Autodesk Fusion 360 part; units mm, degrees
note: some values were not read from the file. Set by a fixed rule: which sketch regions a step uses.
(part 20 of 59)
  spline S113 degree 5 poles (-3.9508, -16.2753) (-3.9508, -16.2754) (-3.9508, -16.2756) (-3.9509, -16.2759) (-3.9509, -16.2764) (-3.951, -16.2772) (-3.9511, -16.278) (-3.9512, -16.279) (-3.9514, -16.2801) (-3.9515, -16.2813) (-3.9517, -16.2826) (-3.9518, -16.284) (-3.952, -16.2855) (-3.9522, -16.2871) (-3.9523, -16.2889) (-3.9525, -16.2907) (-3.9527, -16.2926) (-3.9529, -16.2946) (-3.9531, -16.2968) (-3.9534, -16.299) (-3.9536, -16.3013) (-3.9538, -16.3037) (-3.954, -16.3063) (-3.9543, -16.3089) (-3.9545, -16.3116) (-3.9547, -16.3144) (-3.955, -16.3172) (-3.9552, -16.3202) (-3.9555, -16.3233) (-3.9557, -16.3264) (-3.9559, -16.3297) (-3.9562, -16.333) (-3.9564, -16.3364) (-3.9567, -16.3399) (-3.9569, -16.3435) (-3.9572, -16.3472) (-3.9574, -16.3509) (-3.9577, -16.3547) (-3.9579, -16.3586) (-3.9581, -16.3626) (-3.9584, -16.3667) (-3.9586, -16.3709) (-3.9588, -16.3751) (-3.959, -16.3794) (-3.9593, -16.3838) (-3.9595, -16.3882) (-3.9597, -16.3928) (-3.9599, -16.3974) (-3.9601, -16.4021) (-3.9603, -16.4068) (-3.9605, -16.4117) (-3.9607, -16.4166) (-3.9609, -16.4215) (-3.961, -16.4266) (-3.9612, -16.4317) (-3.9614, -16.4369) (-3.9615, -16.4422) (-3.9617, -16.4475) (-3.9618, -16.4529) (-3.962, -16.4584) (-3.9621, -16.4639) (-3.9622, -16.4695) (-3.9623, -16.4752) (-3.9624, -16.4809) (-3.9625, -16.4867) (-3.9626, -16.4926) (-3.9627, -16.4985) (-3.9627, -16.5045) (-3.9628, -16.5106) (-3.9629, -16.5167) (-3.9629, -16.5229) (-3.9629, -16.5291) (-3.9629, -16.5355) (-3.963, -16.5418) (-3.963, -16.5483) (-3.9629, -16.5548) (-3.9629, -16.5613) (-3.9629, -16.568) (-3.9628, -16.5746) (-3.9628, -16.5814) (-3.9627, -16.5882) (-3.9626, -16.595) (-3.9626, -16.6019) (-3.9625, -16.6089) (-3.9623, -16.6159) (-3.9622, -16.623) (-3.9621, -16.6302) (-3.9619, -16.6374) (-3.9618, -16.6446) (-3.9616, -16.6519) (-3.9614, -16.6593) (-3.9612, -16.6667) (-3.961, -16.6742) (-3.9607, -16.6817) (-3.9605, -16.6893) (-3.9603, -16.697) (-3.96, -16.7047) (-3.9597, -16.7124) (-3.9594, -16.7202) (-3.9591, -16.7281) (-3.9588, -16.736) (-3.9584, -16.7439) (-3.9581, -16.7519) (-3.9577, -16.76) (-3.9573, -16.7681) (-3.9569, -16.7763) (-3.9565, -16.7845) (-3.9561, -16.7927) (-3.9556, -16.801) (-3.9552, -16.8094) (-3.9547, -16.8178) (-3.9542, -16.8263) (-3.9537, -16.8348) (-3.9532, -16.8433) (-3.9526, -16.8519) (-3.9521, -16.8606) (-3.9515, -16.8693) (-3.9509, -16.878) (-3.9503, -16.8868) (-3.9497, -16.8957) (-3.9491, -16.9045) (-3.9484, -16.9135) (-3.9478, -16.9225) (-3.9471, -16.9315) (-3.9464, -16.9406) (-3.9457, -16.9497) (-3.9449, -16.9588) (-3.9442, -16.968) (-3.9434, -16.9773) (-3.9426, -16.9866) (-3.9418, -16.9959) (-3.941, -17.0053) (-3.9402, -17.0147) (-3.9393, -17.0242) (-3.9384, -17.0337) (-3.9375, -17.0433) (-3.9366, -17.0529) (-3.9357, -17.0625) (-3.9348, -17.0722) (-3.9338, -17.0819) (-3.9328, -17.0917) (-3.9318, -17.1015) (-3.9308, -17.1113) (-3.9297, -17.1212) (-3.9287, -17.1312) (-3.9276, -17.1411) (-3.9265, -17.1512) (-3.9254, -17.1612) (-3.9243, -17.1713) (-3.9231, -17.1814) (-3.922, -17.1916) (-3.9208, -17.2018) (-3.9196, -17.2121) (-3.9183, -17.2224) (-3.9171, -17.2327) (-3.9158, -17.2431) (-3.9145, -17.2535) (-3.9132, -17.264) (-3.9119, -17.2744) (-3.9106, -17.285) (-3.9092, -17.2955) (-3.9078, -17.3061) (-3.9064, -17.3168) (-3.905, -17.3274) (-3.9035, -17.3382) (-3.9021, -17.3489) (-3.9006, -17.3597) (-3.8991, -17.3705) (-3.8976, -17.3814) (-3.896, -17.3923) (-3.8945, -17.4032) (-3.8929, -17.4142) (-3.8913, -17.4252) (-3.8896, -17.4362) (-3.888, -17.4473) (-3.8863, -17.4584) (-3.8846, -17.4696) (-3.8829, -17.4807) (-3.8812, -17.492) (-3.8795, -17.5032) (-3.8777, -17.5145) (-3.8759, -17.5258) (-3.8741, -17.5372) (-3.8722, -17.5486) (-3.8704, -17.56) (-3.8685, -17.5714) (-3.8666, -17.5829) (-3.8647, -17.5944) (-3.8628, -17.606) (-3.8608, -17.6176) (-3.8588, -17.6292) (-3.8568, -17.6409) (-3.8548, -17.6525) (-3.8527, -17.6643) (-3.8507, -17.676) (-3.8486, -17.6878) (-3.8464, -17.6996) (-3.8443, -17.7115) (-3.8422, -17.7233) (-3.84, -17.7353) (-3.8378, -17.7472) (-3.8356, -17.7592) (-3.8333, -17.7712) (-3.831, -17.7832) (-3.8288, -17.7953) (-3.8264, -17.8074) (-3.8241, -17.8195) (-3.8217, -17.8317) (-3.8194, -17.8439) (-3.817, -17.8561) (-3.8145, -17.8683) (-3.8121, -17.8806) (-3.8096, -17.8929) (-3.8071, -17.9053) (-3.8046, -17.9176) (-3.8021, -17.93) (-3.7995, -17.9424) (-3.797, -17.9549) (-3.7943, -17.9674) (-3.7917, -17.9799) (-3.7891, -17.9924) (-3.7864, -18.005) (-3.7837, -18.0176) (-3.781, -18.0302) (-3.7782, -18.0429) (-3.7755, -18.0556) (-3.7727, -18.0683) (-3.7699, -18.081) (-3.767, -18.0938) (-3.7642, -18.1066) (-3.7613, -18.1194) (-3.7584, -18.1323) (-3.7555, -18.1451) (-3.7525, -18.158) (-3.7496, -18.171) (-3.7466, -18.1839) (-3.7435, -18.1969) (-3.7405, -18.2099) (-3.7374, -18.223) (-3.7343, -18.236) (-3.7312, -18.2491) (-3.7287, -18.2596) (-3.7268, -18.2675) (-3.7256, -18.2728) (-3.7249, -18.2754) knots 0 0 0 0 0 0 0.00416667 0.00833333 0.0125 0.01666667 0.02083333 0.025 0.02916667 0.03333333 0.0375 0.04166667 0.04583333 0.05 0.05416667 0.05833333 0.0625 0.06666667 0.07083333 0.075 0.07916667 0.08333333 0.0875 0.09166667 0.09583333 0.1 0.10416667 0.10833333 0.1125 0.11666667 0.12083333 0.125 0.12916667 0.13333333 0.1375 0.14166667 0.14583333 0.15 0.15416667 0.15833333 0.1625 0.16666667 0.17083333 0.175 0.17916667 0.18333333 0.1875 0.19166667 0.19583333 0.2 0.20416667 0.20833333 0.2125 0.21666667 0.22083333 0.225 0.22916667 0.23333333 0.2375 0.24166667 0.24583333 0.25 0.25416667 0.25833333 0.2625 0.26666667 0.27083333 0.275 0.27916667 0.28333333 0.2875 0.29166667 0.29583333 0.3 0.30416667 0.30833333 0.3125 0.31666667 0.32083333 0.325 0.32916667 0.33333333 0.3375 0.34166667 0.34583333 0.35 0.35416667 0.35833333 0.3625 0.36666667 0.37083333 0.375 0.37916667 0.38333333 0.3875 0.39166667 0.39583333 0.4 0.40416667 0.40833333 0.4125 0.41666667 0.42083333 0.425 0.42916667 0.43333333 0.4375 0.44166667 0.44583333 0.45 0.45416667 0.45833333 0.4625 0.46666667 0.47083333 0.475 0.47916667 0.48333333 0.4875 0.49166667 0.49583333 0.5 0.50416667 0.50833333 0.5125 0.51666667 0.52083333 0.525 0.52916667 0.53333333 0.5375 0.54166667 0.54583333 0.55 0.55416667 0.55833333 0.5625 0.56666667 0.57083333 0.575 0.57916667 0.58333333 0.5875 0.59166667 0.59583333 0.6 0.60416667 0.60833333 0.6125 0.61666667 0.62083333 0.625 0.62916667 0.63333333 0.6375 0.64166667 0.64583333 0.65 0.65416667 0.65833333 0.6625 0.66666667 0.67083333 0.675 0.67916667 0.68333333 0.6875 0.69166667 0.69583333 0.7 0.70416667 0.70833333 0.7125 0.71666667 0.72083333 0.725 0.72916667 0.73333333 0.7375 0.74166667 0.74583333 0.75 0.75416667 0.75833333 0.7625 0.76666667 0.77083333 0.775 0.77916667 0.78333333 0.7875 0.79166667 0.79583333 0.8 0.80416667 0.80833333 0.8125 0.81666667 0.82083333 0.825 0.82916667 0.83333333 0.8375 0.84166667 0.84583333 0.85 0.85416667 0.85833333 0.8625 0.86666667 0.87083333 0.875 0.87916667 0.88333333 0.8875 0.89166667 0.89583333 0.9 0.90416667 0.90833333 0.9125 0.91666667 0.92083333 0.925 0.92916667 0.93333333 0.9375 0.94166667 0.94583333 0.95 0.95416667 0.95833333 0.9625 0.96666667 0.97083333 0.975 0.97916667 0.98333333 0.9875 0.99166667 0.99583333 1 1 1 1 1 1
  line L242 (18.7406, 34.6904) -> (18.7401, 34.6898)
  line L243 (3.9507, 41.2745) -> (3.9508, 41.2753)
  spline S114 degree 5 poles (8.0948, -15.3945) (8.0948, -15.3946) (8.0948, -15.3948) (8.0949, -15.3951) (8.0951, -15.3956) (8.0953, -15.3963) (8.0956, -15.3971) (8.0958, -15.398) (8.0962, -15.3991) (8.0965, -15.4002) (8.0969, -15.4015) (8.0973, -15.4028) (8.0978, -15.4043) (8.0983, -15.4058) (8.0988, -15.4075) (8.0994, -15.4092) (8.1, -15.4111) (8.1007, -15.413) (8.1013, -15.415) (8.102, -15.4172) (8.1028, -15.4194) (8.1036, -15.4217) (8.1044, -15.4241) (8.1052, -15.4265) (8.1061, -15.4291) (8.107, -15.4318) (8.108, -15.4345) (8.109, -15.4373) (8.11, -15.4402) (8.1111, -15.4432) (8.1121, -15.4462) (8.1133, -15.4494) (8.1144, -15.4526) (8.1156, -15.4559) (8.1169, -15.4593) (8.1181, -15.4627) (8.1194, -15.4662) (8.1208, -15.4698) (8.1222, -15.4735) (8.1236, -15.4772) (8.125, -15.4811) (8.1265, -15.4849) (8.128, -15.4889) (8.1295, -15.4929) (8.1311, -15.497) (8.1327, -15.5012) (8.1344, -15.5054) (8.1361, -15.5097) (8.1378, -15.5141) (8.1395, -15.5185) (8.1413, -15.523) (8.1432, -15.5276) (8.145, -15.5322) (8.1469, -15.5369) (8.1488, -15.5416) (8.1508, -15.5464) (8.1528, -15.5513) (8.1548, -15.5562) (8.1569, -15.5612) (8.159, -15.5663) (8.1611, -15.5714) (8.1633, -15.5765) (8.1655, -15.5818) (8.1677, -15.587) (8.17, -15.5924) (8.1723, -15.5978) (8.1747, -15.6032) (8.177, -15.6087) (8.1795, -15.6143) (8.1819, -15.6199) (8.1844, -15.6256) (8.1869, -15.6313) (8.1895, -15.6371) (8.192, -15.6429) (8.1947, -15.6488) (8.1973, -15.6547) (8.2, -15.6607) (8.2027, -15.6667) (8.2055, -15.6728) (8.2083, -15.679) (8.2111, -15.6851) (8.214, -15.6914) (8.2169, -15.6977) (8.2198, -15.704) (8.2227, -15.7104) (8.2257, -15.7168) (8.2288, -15.7233) (8.2318, -15.7298) (8.2349, -15.7363) (8.2381, -15.7429) (8.2412, -15.7496) (8.2445, -15.7563) (8.2477, -15.763) (8.251, -15.7698) (8.2543, -15.7767) (8.2576, -15.7835) (8.261, -15.7905) (8.2644, -15.7974) (8.2678, -15.8044) (8.2713, -15.8115) (8.2748, -15.8186) (8.2784, -15.8257) (8.282, -15.8329) (8.2856, -15.8401) (8.2892, -15.8473) (8.2929, -15.8546) (8.2966, -15.8619) (8.3004, -15.8693) (8.3042, -15.8767) (8.308, -15.8842) (8.3118, -15.8917) (8.3157, -15.8992) (8.3196, -15.9068) (8.3236, -15.9144) (8.3276, -15.922) (8.3316, -15.9297) (8.3357, -15.9374) (8.3398, -15.9452) (8.3439, -15.9529) (8.348, -15.9608) (8.3522, -15.9686) (8.3565, -15.9765) (8.3607, -15.9845) (8.365, -15.9924) (8.3693, -16.0004) (8.3737, -16.0085) (8.3781, -16.0165) (8.3825, -16.0246) (8.387, -16.0328) (8.3915, -16.0409) (8.396, -16.0491) (8.4006, -16.0574) (8.4052, -16.0657) (8.4098, -16.074) (8.4145, -16.0823) (8.4192, -16.0907) (8.4239, -16.0991) (8.4287, -16.1075) (8.4335, -16.116) (8.4384, -16.1244) (8.4432, -16.133) (8.4481, -16.1415) (8.4531, -16.1501) (8.458, -16.1587) (8.463, -16.1674) (8.4681, -16.176) (8.4732, -16.1847) (8.4783, -16.1935) (8.4834, -16.2022) (8.4886, -16.211) (8.4938, -16.2199) (8.499, -16.2287) (8.5043, -16.2376) (8.5096, -16.2465) (8.515, -16.2554) (8.5203, -16.2644) (8.5257, -16.2734) (8.5312, -16.2824) (8.5367, -16.2914) (8.5422, -16.3005) (8.5477, -16.3096) (8.5533, -16.3187) (8.5589, -16.3279) (8.5645, -16.337) (8.5702, -16.3462) (8.5759, -16.3555) (8.5817, -16.3647) (8.5874, -16.374) (8.5932, -16.3833) (8.5991, -16.3926) (8.605, -16.402) (8.6109, -16.4113) (8.6168, -16.4207) (8.6228, -16.4302) (8.6288, -16.4396) (8.6348, -16.4491) (8.6409, -16.4586) (8.647, -16.4681) (8.6532, -16.4776) (8.6593, -16.4872) (8.6656, -16.4968) (8.6718, -16.5064) (8.6781, -16.516) (8.6844, -16.5257) (8.6907, -16.5354) (8.6971, -16.5451) (8.7035, -16.5548) (8.7099, -16.5646) (8.7164, -16.5743) (8.7229, -16.5841) (8.7295, -16.5939) (8.736, -16.6037) (8.7426, -16.6136) (8.7493, -16.6235) (8.7559, -16.6334) (8.7626, -16.6433) (8.7694, -16.6532) (8.7762, -16.6632) (8.783, -16.6731) (8.7898, -16.6831) (8.7967, -16.6932) (8.8036, -16.7032) (8.8105, -16.7132) (8.8175, -16.7233) (8.8245, -16.7334) (8.8315, -16.7435) (8.8386, -16.7537) (8.8457, -16.7638) (8.8528, -16.774) (8.86, -16.7842) (8.8671, -16.7944) (8.8744, -16.8046) (8.8816, -16.8148) (8.8889, -16.8251) (8.8963, -16.8354) (8.9036, -16.8457) (8.911, -16.856) (8.9184, -16.8663) (8.9259, -16.8766) (8.9334, -16.887) (8.9409, -16.8974) (8.9485, -16.9078) (8.956, -16.9182) (8.9637, -16.9286) (8.9713, -16.9391) (8.979, -16.9495) (8.9867, -16.96) (8.9945, -16.9705) (9.0022, -16.981) (9.0101, -16.9915) (9.0179, -17.0021) (9.0258, -17.0127) (9.0337, -17.0232) (9.0416, -17.0338) (9.0496, -17.0444) (9.0576, -17.055) (9.0657, -17.0657) (9.0737, -17.0763) (9.0818, -17.087) (9.09, -17.0977) (9.0981, -17.1084) (9.1047, -17.1169) (9.1096, -17.1234) (9.1129, -17.1276) (9.1146, -17.1298) knots 0 0 0 0 0 0 0.00416667 0.00833333 0.0125 0.01666667 0.02083333 0.025 0.02916667 0.03333333 0.0375 0.04166667 0.04583333 0.05 0.05416667 0.05833333 0.0625 0.06666667 0.07083333 0.075 0.07916667 0.08333333 0.0875 0.09166667 0.09583333 0.1 0.10416667 0.10833333 0.1125 0.11666667 0.12083333 0.125 0.12916667 0.13333333 0.1375 0.14166667 0.14583333 0.15 0.15416667 0.15833333 0.1625 0.16666667 0.17083333 0.175 0.17916667 0.18333333 0.1875 0.19166667 0.19583333 0.2 0.20416667 0.20833333 0.2125 0.21666667 0.22083333 0.225 0.22916667 0.23333333 0.2375 0.24166667 0.24583333 0.25 0.25416667 0.25833333 0.2625 0.26666667 0.27083333 0.275 0.27916667 0.28333333 0.2875 0.29166667 0.29583333 0.3 0.30416667 0.30833333 0.3125 0.31666667 0.32083333 0.325 0.32916667 0.33333333 0.3375 0.34166667 0.34583333 0.35 0.35416667 0.35833333 0.3625 0.36666667 0.37083333 0.375 0.37916667 0.38333333 0.3875 0.39166667 0.39583333 0.4 0.40416667 0.40833333 0.4125 0.41666667 0.42083333 0.425 0.42916667 0.43333333 0.4375 0.44166667 0.44583333 0.45 0.45416667 0.45833333 0.4625 0.46666667 0.47083333 0.475 0.47916667 0.48333333 0.4875 0.49166667 0.49583333 0.5 0.50416667 0.50833333 0.5125 0.51666667 0.52083333 0.525 0.52916667 0.53333333 0.5375 0.54166667 0.54583333 0.55 0.55416667 0.55833333 0.5625 0.56666667 0.57083333 0.575 0.57916667 0.58333333 0.5875 0.59166667 0.59583333 0.6 0.60416667 0.60833333 0.6125 0.61666667 0.62083333 0.625 0.62916667 0.63333333 0.6375 0.64166667 0.64583333 0.65 0.65416667 0.65833333 0.6625 0.66666667 0.67083333 0.675 0.67916667 0.68333333 0.6875 0.69166667 0.69583333 0.7 0.70416667 0.70833333 0.7125 0.71666667 0.72083333 0.725 0.72916667 0.73333333 0.7375 0.74166667 0.74583333 0.75 0.75416667 0.75833333 0.7625 0.76666667 0.77083333 0.775 0.77916667 0.78333333 0.7875 0.79166667 0.79583333 0.8 0.80416667 0.80833333 0.8125 0.81666667 0.82083333 0.825 0.82916667 0.83333333 0.8375 0.84166667 0.84583333 0.85 0.85416667 0.85833333 0.8625 0.86666667 0.87083333 0.875 0.87916667 0.88333333 0.8875 0.89166667 0.89583333 0.9 0.90416667 0.90833333 0.9125 0.91666667 0.92083333 0.925 0.92916667 0.93333333 0.9375 0.94166667 0.94583333 0.95 0.95416667 0.95833333 0.9625 0.96666667 0.97083333 0.975 0.97916667 0.98333333 0.9875 0.99166667 0.99583333 1 1 1 1 1 1
  arc A121 (-5.0824, -15.7972) -> (-3.9106, -15.9828) centre (0, 12.5) ccw
  line L244 (28.587, 17.6345) -> (28.5878, 17.6346)
  spline S115 degree 5 poles (6.937, 40.7047) (6.937, 40.7048) (6.937, 40.705) (6.9371, 40.7053) (6.9372, 40.7058) (6.9374, 40.7065) (6.9376, 40.7074) (6.9378, 40.7083) (6.9381, 40.7094) (6.9383, 40.7106) (6.9386, 40.7118) (6.9389, 40.7132) (6.9392, 40.7147) (6.9396, 40.7163) (6.9399, 40.718) (6.9403, 40.7198) (6.9407, 40.7217) (6.9411, 40.7237) (6.9416, 40.7258) (6.942, 40.728) (6.9425, 40.7303) (6.9429, 40.7327) (6.9434, 40.7351) (6.9439, 40.7377) (6.9445, 40.7404) (6.945, 40.7431) (6.9455, 40.746) (6.9461, 40.7489) (6.9466, 40.7519) (6.9472, 40.755) (6.9478, 40.7582) (6.9484, 40.7615) (6.949, 40.7649) (6.9496, 40.7683) (6.9502, 40.7719) (6.9508, 40.7755) (6.9515, 40.7792) (6.9521, 40.783) (6.9528, 40.7868) (6.9534, 40.7908) (6.9541, 40.7948) (6.9547, 40.7989) (6.9554, 40.8031) (6.9561, 40.8074) (6.9568, 40.8117) (6.9574, 40.8161) (6.9581, 40.8206) (6.9588, 40.8252) (6.9595, 40.8298) (6.9602, 40.8345) (6.9609, 40.8393) (6.9616, 40.8442) (6.9623, 40.8491) (6.963, 40.8541) (6.9637, 40.8592) (6.9644, 40.8643) (6.9651, 40.8695) (6.9658, 40.8748) (6.9665, 40.8802) (6.9672, 40.8856) (6.9679, 40.8911) (6.9686, 40.8966) (6.9693, 40.9023) (6.97, 40.908) (6.9707, 40.9137) (6.9714, 40.9196) (6.9721, 40.9255) (6.9728, 40.9314) (6.9735, 40.9374) (6.9742, 40.9435) (6.9749, 40.9497) (6.9756, 40.9559) (6.9763, 40.9622) (6.9769, 40.9685) (6.9776, 40.9749) (6.9783, 40.9814) (6.9789, 40.9879) (6.9796, 40.9945) (6.9803, 41.0011) (6.9809, 41.0078) (6.9816, 41.0146) (6.9822, 41.0214) (6.9828, 41.0283) (6.9835, 41.0353) (6.9841, 41.0423) (6.9847, 41.0493) (6.9853, 41.0564) (6.9859, 41.0636) (6.9865, 41.0709) (6.9871, 41.0781) (6.9877, 41.0855) (6.9882, 41.0929) (6.9888, 41.1004) (6.9894, 41.1079) (6.9899, 41.1154) (6.9905, 41.1231) (6.991, 41.1307) (6.9915, 41.1385) (6.9921, 41.1463) (6.9926, 41.1541) (6.9931, 41.162) (6.9936, 41.17) (6.994, 41.178) (6.9945, 41.186) (6.995, 41.1941) (6.9954, 41.2023) (6.9959, 41.2105) (6.9963, 41.2187) (6.9968, 41.227) (6.9972, 41.2354) (6.9976, 41.2438) (6.998, 41.2523) (6.9984, 41.2608) (6.9987, 41.2694) (6.9991, 41.278) (6.9995, 41.2866) (6.9998, 41.2953) (7.0001, 41.3041) (7.0005, 41.3129) (7.0008, 41.3218) (7.0011, 41.3307) (7.0014, 41.3396) (7.0016, 41.3486) (7.0019, 41.3577) (7.0021, 41.3668) (7.0024, 41.3759) (7.0026, 41.3851) (7.0028, 41.3943) (7.003, 41.4036) (7.0032, 41.4129) (7.0034, 41.4223) (7.0036, 41.4317) (7.0037, 41.4412) (7.0038, 41.4507) (7.004, 41.4602) (7.0041, 41.4698) (7.0042, 41.4795) (7.0043, 41.4892) (7.0043, 41.4989) (7.0044, 41.5087) (7.0044, 41.5185) (7.0045, 41.5284) (7.0045, 41.5383) (7.0045, 41.5482) (7.0045, 41.5582) (7.0044, 41.5682) (7.0044, 41.5783) (7.0043, 41.5884) (7.0043, 41.5986) (7.0042, 41.6088) (7.0041, 41.619) (7.004, 41.6293) (7.0038, 41.6396) (7.0037, 41.65) (7.0035, 41.6604) (7.0034, 41.6708) (7.0032, 41.6813) (7.003, 41.6919) (7.0028, 41.7024) (7.0025, 41.713) (7.0023, 41.7237) (7.002, 41.7344) (7.0017, 41.7451) (7.0014, 41.7559) (7.0011, 41.7667) (7.0008, 41.7775) (7.0004, 41.7884) (7.0001, 41.7993) (6.9997, 41.8103) (6.9993, 41.8213) (6.9989, 41.8323) (6.9984, 41.8434) (6.998, 41.8545) (6.9975, 41.8657) (6.997, 41.8768) (6.9965, 41.8881) (6.996, 41.8993) (6.9955, 41.9106) (6.995, 41.922) (6.9944, 41.9333) (6.9938, 41.9447) (6.9932, 41.9562) (6.9926, 41.9677) (6.992, 41.9792) (6.9913, 41.9907) (6.9906, 42.0023) (6.99, 42.014) (6.9892, 42.0256) (6.9885, 42.0373) (6.9878, 42.049) (6.987, 42.0608) (6.9863, 42.0726) (6.9855, 42.0844) (6.9846, 42.0963) (6.9838, 42.1082) (6.983, 42.1201) (6.9821, 42.1321) (6.9812, 42.1441) (6.9803, 42.1562) (6.9794, 42.1682) (6.9784, 42.1803) (6.9775, 42.1925) (6.9765, 42.2047) (6.9755, 42.2169) (6.9745, 42.2291) (6.9735, 42.2414) (6.9724, 42.2537) (6.9713, 42.266) (6.9702, 42.2784) (6.9691, 42.2908) (6.968, 42.3032) (6.9669, 42.3157) (6.9657, 42.3282) (6.9645, 42.3407) (6.9633, 42.3533) (6.9621, 42.3659) (6.9608, 42.3785) (6.9596, 42.3912) (6.9583, 42.4039) (6.957, 42.4166) (6.9556, 42.4293) (6.9543, 42.4421) (6.9529, 42.4549) (6.9516, 42.4678) (6.9501, 42.4806) (6.9487, 42.4935) (6.9473, 42.5065) (6.9458, 42.5194) (6.9443, 42.5324) (6.9428, 42.5455) (6.9413, 42.5585) (6.9398, 42.5716) (6.9382, 42.5847) (6.9366, 42.5979) (6.935, 42.611) (6.9334, 42.6242) (6.9317, 42.6375) (6.9301, 42.6507) (6.9284, 42.664) (6.9267, 42.6773) (6.925, 42.6907) (6.9236, 42.7014) (6.9225, 42.7094) (6.9218, 42.7148) (6.9214, 42.7174) knots 0 0 0 0 0 0 0.00416667 0.00833333 0.0125 0.01666667 0.02083333 0.025 0.02916667 0.03333333 0.0375 0.04166667 0.04583333 0.05 0.05416667 0.05833333 0.0625 0.06666667 0.07083333 0.075 0.07916667 0.08333333 0.0875 0.09166667 0.09583333 0.1 0.10416667 0.10833333 0.1125 0.11666667 0.12083333 0.125 0.12916667 0.13333333 0.1375 0.14166667 0.14583333 0.15 0.15416667 0.15833333 0.1625 0.16666667 0.17083333 0.175 0.17916667 0.18333333 0.1875 0.19166667 0.19583333 0.2 0.20416667 0.20833333 0.2125 0.21666667 0.22083333 0.225 0.22916667 0.23333333 0.2375 0.24166667 0.24583333 0.25 0.25416667 0.25833333 0.2625 0.26666667 0.27083333 0.275 0.27916667 0.28333333 0.2875 0.29166667 0.29583333 0.3 0.30416667 0.30833333 0.3125 0.31666667 0.32083333 0.325 0.32916667 0.33333333 0.3375 0.34166667 0.34583333 0.35 0.35416667 0.35833333 0.3625 0.36666667 0.37083333 0.375 0.37916667 0.38333333 0.3875 0.39166667 0.39583333 0.4 0.40416667 0.40833333 0.4125 0.41666667 0.42083333 0.425 0.42916667 0.43333333 0.4375 0.44166667 0.44583333 0.45 0.45416667 0.45833333 0.4625 0.46666667 0.47083333 0.475 0.47916667 0.48333333 0.4875 0.49166667 0.49583333 0.5 0.50416667 0.50833333 0.5125 0.51666667 0.52083333 0.525 0.52916667 0.53333333 0.5375 0.54166667 0.54583333 0.55 0.55416667 0.55833333 0.5625 0.56666667 0.57083333 0.575 0.57916667 0.58333333 0.5875 0.59166667 0.59583333 0.6 0.60416667 0.60833333 0.6125 0.61666667 0.62083333 0.625 0.62916667 0.63333333 0.6375 0.64166667 0.64583333 0.65 0.65416667 0.65833333 0.6625 0.66666667 0.67083333 0.675 0.67916667 0.68333333 0.6875 0.69166667 0.69583333 0.7 0.70416667 0.70833333 0.7125 0.71666667 0.72083333 0.725 0.72916667 0.73333333 0.7375 0.74166667 0.74583333 0.75 0.75416667 0.75833333 0.7625 0.76666667 0.77083333 0.775 0.77916667 0.78333333 0.7875 0.79166667 0.79583333 0.8 0.80416667 0.80833333 0.8125 0.81666667 0.82083333 0.825 0.82916667 0.83333333 0.8375 0.84166667 0.84583333 0.85 0.85416667 0.85833333 0.8625 0.86666667 0.87083333 0.875 0.87916667 0.88333333 0.8875 0.89166667 0.89583333 0.9 0.90416667 0.90833333 0.9125 0.91666667 0.92083333 0.925 0.92916667 0.93333333 0.9375 0.94166667 0.94583333 0.95 0.95416667 0.95833333 0.9625 0.96666667 0.97083333 0.975 0.97916667 0.98333333 0.9875 0.99166667 0.99583333 1 1 1 1 1 1
  spline S116 degree 5 poles (29.0307, 11.5787) (29.0307, 11.5787) (29.0309, 11.5787) (29.0313, 11.5787) (29.0318, 11.5787) (29.0325, 11.5787) (29.0334, 11.5787) (29.0344, 11.5786) (29.0355, 11.5786) (29.0367, 11.5786) (29.038, 11.5786) (29.0394, 11.5786) (29.0409, 11.5786) (29.0425, 11.5786) (29.0443, 11.5786) (29.0461, 11.5786) (29.0481, 11.5786) (29.0501, 11.5786) (29.0522, 11.5786) (29.0545, 11.5786) (29.0568, 11.5786) (29.0592, 11.5787) (29.0618, 11.5787) (29.0644, 11.5788) (29.0671, 11.5788) (29.0699, 11.5789) (29.0728, 11.5789) (29.0758, 11.579) (29.0788, 11.5791) (29.082, 11.5792) (29.0852, 11.5792) (29.0886, 11.5794) (29.092, 11.5795) (29.0955, 11.5796) (29.0991, 11.5797) (29.1028, 11.5799) (29.1065, 11.58) (29.1103, 11.5802) (29.1143, 11.5803) (29.1183, 11.5805) (29.1223, 11.5807) (29.1265, 11.5809) (29.1307, 11.5811) (29.135, 11.5814) (29.1394, 11.5816) (29.1439, 11.5818) (29.1484, 11.5821) (29.153, 11.5824) (29.1577, 11.5827) (29.1624, 11.583) (29.1673, 11.5833) (29.1722, 11.5836) (29.1771, 11.5839) (29.1822, 11.5843) (29.1873, 11.5847) (29.1925, 11.585) (29.1977, 11.5854) (29.203, 11.5859) (29.2084, 11.5863) (29.2139, 11.5867) (29.2194, 11.5872) (29.225, 11.5876) (29.2306, 11.5881) (29.2363, 11.5886) (29.2421, 11.5891) (29.248, 11.5897) (29.2539, 11.5902) (29.2599, 11.5908) (29.2659, 11.5913) (29.272, 11.5919) (29.2781, 11.5925) (29.2844, 11.5932) (29.2906, 11.5938) (29.297, 11.5945) (29.3034, 11.5951) (29.3099, 11.5958) (29.3164, 11.5965) (29.323, 11.5973) (29.3296, 11.598) (29.3363, 11.5988) (29.343, 11.5995) (29.3498, 11.6003) (29.3567, 11.6011) (29.3636, 11.602) (29.3706, 11.6028) (29.3777, 11.6037) (29.3847, 11.6046) (29.3919, 11.6055) (29.3991, 11.6064) (29.4063, 11.6073) (29.4137, 11.6083) (29.421, 11.6093) (29.4284, 11.6103) (29.4359, 11.6113) (29.4434, 11.6123) (29.451, 11.6134) (29.4586, 11.6144) (29.4663, 11.6155) (29.474, 11.6166) (29.4818, 11.6178) (29.4896, 11.6189) (29.4975, 11.6201) (29.5054, 11.6213) (29.5134, 11.6225) (29.5214, 11.6237) (29.5295, 11.625) (29.5376, 11.6262) (29.5458, 11.6275) (29.554, 11.6288) (29.5623, 11.6302) (29.5706, 11.6315) (29.5789, 11.6329) (29.5873, 11.6343) (29.5958, 11.6357) (29.6043, 11.6371) (29.6128, 11.6386) (29.6214, 11.64) (29.6301, 11.6415) (29.6388, 11.6431) (29.6475, 11.6446) (29.6563, 11.6462) (29.6651, 11.6477) (29.6739, 11.6493) (29.6828, 11.651) (29.6918, 11.6526) (29.7008, 11.6543) (29.7098, 11.656) (29.7189, 11.6577) (29.728, 11.6594) (29.7372, 11.6612) (29.7464, 11.6629) (29.7556, 11.6647) (29.7649, 11.6666) (29.7742, 11.6684) (29.7836, 11.6703) (29.793, 11.6721) (29.8025, 11.6741) (29.812, 11.676) (29.8215, 11.6779) (29.8311, 11.6799) (29.8407, 11.6819) (29.8503, 11.6839) (29.86, 11.686) (29.8697, 11.688) (29.8795, 11.6901) (29.8893, 11.6922) (29.8992, 11.6944) (29.909, 11.6965) (29.919, 11.6987) (29.9289, 11.7009) (29.9389, 11.7031) (29.949, 11.7054) (29.959, 11.7077) (29.9691, 11.71) (29.9793, 11.7123) (29.9895, 11.7146) (29.9997, 11.717) (30.0099, 11.7194) (30.0202, 11.7218) (30.0306, 11.7242) (30.0409, 11.7267) (30.0513, 11.7292) (30.0618, 11.7317) (30.0722, 11.7342) (30.0827, 11.7368) (30.0933, 11.7394) (30.1038, 11.742) (30.1145, 11.7446) (30.1251, 11.7472) (30.1358, 11.7499) (30.1465, 11.7526) (30.1572, 11.7553) (30.168, 11.7581) (30.1788, 11.7609) (30.1897, 11.7636) (30.2005, 11.7665) (30.2114, 11.7693) (30.2224, 11.7722) (30.2334, 11.7751) (30.2444, 11.778) (30.2554, 11.7809) (30.2665, 11.7839) (30.2776, 11.7869) (30.2887, 11.7899) (30.2999, 11.7929) (30.3111, 11.796) (30.3223, 11.7991) (30.3336, 11.8022) (30.3448, 11.8053) (30.3562, 11.8085) (30.3675, 11.8117) (30.3789, 11.8149) (30.3903, 11.8181) (30.4017, 11.8214) (30.4132, 11.8247) (30.4247, 11.828) (30.4362, 11.8313) (30.4478, 11.8347) (30.4594, 11.8381) (30.471, 11.8415) (30.4827, 11.8449) (30.4943, 11.8484) (30.506, 11.8519) (30.5178, 11.8554) (30.5295, 11.8589) (30.5413, 11.8625) (30.5531, 11.8661) (30.565, 11.8697) (30.5769, 11.8733) (30.5888, 11.877) (30.6007, 11.8807) (30.6126, 11.8844) (30.6246, 11.8882) (30.6366, 11.8919) (30.6487, 11.8957) (30.6607, 11.8995) (30.6728, 11.9034) (30.685, 11.9073) (30.6971, 11.9111) (30.7093, 11.9151) (30.7215, 11.919) (30.7337, 11.923) (30.7459, 11.927) (30.7582, 11.931) (30.7705, 11.9351) (30.7828, 11.9391) (30.7952, 11.9432) (30.8076, 11.9474) (30.82, 11.9515) (30.8324, 11.9557) (30.8448, 11.9599) (30.8573, 11.9641) (30.8698, 11.9684) (30.8823, 11.9727) (30.8949, 11.977) (30.9075, 11.9813) (30.9201, 11.9857) (30.9327, 11.9901) (30.9453, 11.9945) (30.958, 11.9989) (30.9707, 12.0034) (30.9809, 12.007) (30.9885, 12.0097) (30.9936, 12.0115) (30.9962, 12.0124) knots 0 0 0 0 0 0 0.00416667 0.00833333 0.0125 0.01666667 0.02083333 0.025 0.02916667 0.03333333 0.0375 0.04166667 0.04583333 0.05 0.05416667 0.05833333 0.0625 0.06666667 0.07083333 0.075 0.07916667 0.08333333 0.0875 0.09166667 0.09583333 0.1 0.10416667 0.10833333 0.1125 0.11666667 0.12083333 0.125 0.12916667 0.13333333 0.1375 0.14166667 0.14583333 0.15 0.15416667 0.15833333 0.1625 0.16666667 0.17083333 0.175 0.17916667 0.18333333 0.1875 0.19166667 0.19583333 0.2 0.20416667 0.20833333 0.2125 0.21666667 0.22083333 0.225 0.22916667 0.23333333 0.2375 0.24166667 0.24583333 0.25 0.25416667 0.25833333 0.2625 0.26666667 0.27083333 0.275 0.27916667 0.28333333 0.2875 0.29166667 0.29583333 0.3 0.30416667 0.30833333 0.3125 0.31666667 0.32083333 0.325 0.32916667 0.33333333 0.3375 0.34166667 0.34583333 0.35 0.35416667 0.35833333 0.3625 0.36666667 0.37083333 0.375 0.37916667 0.38333333 0.3875 0.39166667 0.39583333 0.4 0.40416667 0.40833333 0.4125 0.41666667 0.42083333 0.425 0.42916667 0.43333333 0.4375 0.44166667 0.44583333 0.45 0.45416667 0.45833333 0.4625 0.46666667 0.47083333 0.475 0.47916667 0.48333333 0.4875 0.49166667 0.49583333 0.5 0.50416667 0.50833333 0.5125 0.51666667 0.52083333 0.525 0.52916667 0.53333333 0.5375 0.54166667 0.54583333 0.55 0.55416667 0.55833333 0.5625 0.56666667 0.57083333 0.575 0.57916667 0.58333333 0.5875 0.59166667 0.59583333 0.6 0.60416667 0.60833333 0.6125 0.61666667 0.62083333 0.625 0.62916667 0.63333333 0.6375 0.64166667 0.64583333 0.65 0.65416667 0.65833333 0.6625 0.66666667 0.67083333 0.675 0.67916667 0.68333333 0.6875 0.69166667 0.69583333 0.7 0.70416667 0.70833333 0.7125 0.71666667 0.72083333 0.725 0.72916667 0.73333333 0.7375 0.74166667 0.74583333 0.75 0.75416667 0.75833333 0.7625 0.76666667 0.77083333 0.775 0.77916667 0.78333333 0.7875 0.79166667 0.79583333 0.8 0.80416667 0.80833333 0.8125 0.81666667 0.82083333 0.825 0.82916667 0.83333333 0.8375 0.84166667 0.84583333 0.85 0.85416667 0.85833333 0.8625 0.86666667 0.87083333 0.875 0.87916667 0.88333333 0.8875 0.89166667 0.89583333 0.9 0.90416667 0.90833333 0.9125 0.91666667 0.92083333 0.925 0.92916667 0.93333333 0.9375 0.94166667 0.94583333 0.95 0.95416667 0.95833333 0.9625 0.96666667 0.97083333 0.975 0.97916667 0.98333333 0.9875 0.99166667 0.99583333 1 1 1 1 1 1
  arc A122 (8.0125, 40.1109) -> (6.8665, 40.418) centre (0, 12.5) ccw
  arc A123 (-3.7249, -18.2754) -> (-2.755, -18.3773) centre (0, 12.5) ccw
  line L245 (28.2039, 5.5632) -> (28.2047, 5.563)
  arc A124 (-0.4876, -18.4962) -> (0.4876, -18.4962) centre (0, 12.5) ccw
  spline S117 degree 5 poles (9.1146, 42.1298) (9.1129, 42.1276) (9.1096, 42.1234) (9.1047, 42.1169) (9.0981, 42.1084) (9.09, 42.0977) (9.0818, 42.087) (9.0737, 42.0763) (9.0657, 42.0657) (9.0576, 42.055) (9.0496, 42.0444) (9.0416, 42.0338) (9.0337, 42.0232) (9.0258, 42.0127) (9.0179, 42.0021) (9.0101, 41.9915) (9.0022, 41.981) (8.9945, 41.9705) (8.9867, 41.96) (8.979, 41.9495) (8.9713, 41.9391) (8.9637, 41.9286) (8.956, 41.9182) (8.9485, 41.9078) (8.9409, 41.8974) (8.9334, 41.887) (8.9259, 41.8766) (8.9184, 41.8663) (8.911, 41.856) (8.9036, 41.8457) (8.8963, 41.8354) (8.8889, 41.8251) (8.8816, 41.8148) (8.8744, 41.8046) (8.8671, 41.7944) (8.86, 41.7842) (8.8528, 41.774) (8.8457, 41.7638) (8.8386, 41.7537) (8.8315, 41.7435) (8.8245, 41.7334) (8.8175, 41.7233) (8.8105, 41.7132) (8.8036, 41.7032) (8.7967, 41.6932) (8.7898, 41.6831) (8.783, 41.6731) (8.7762, 41.6632) (8.7694, 41.6532) (8.7626, 41.6433) (8.7559, 41.6334) (8.7493, 41.6235) (8.7426, 41.6136) (8.736, 41.6037) (8.7295, 41.5939) (8.7229, 41.5841) (8.7164, 41.5743) (8.7099, 41.5646) (8.7035, 41.5548) (8.6971, 41.5451) (8.6907, 41.5354) (8.6844, 41.5257) (8.6781, 41.516) (8.6718, 41.5064) (8.6656, 41.4968) (8.6593, 41.4872) (8.6532, 41.4776) (8.647, 41.4681) (8.6409, 41.4586) (8.6348, 41.4491) (8.6288, 41.4396) (8.6228, 41.4302) (8.6168, 41.4207) (8.6109, 41.4113) (8.605, 41.402) (8.5991, 41.3926) (8.5932, 41.3833) (8.5874, 41.374) (8.5817, 41.3647) (8.5759, 41.3555) (8.5702, 41.3462) (8.5645, 41.337) (8.5589, 41.3279) (8.5533, 41.3187) (8.5477, 41.3096) (8.5422, 41.3005) (8.5367, 41.2914) (8.5312, 41.2824) (8.5257, 41.2734) (8.5203, 41.2644) (8.515, 41.2554) (8.5096, 41.2465) (8.5043, 41.2376) (8.499, 41.2287) (8.4938, 41.2199) (8.4886, 41.211) (8.4834, 41.2022) (8.4783, 41.1935) (8.4732, 41.1847) (8.4681, 41.176) (8.463, 41.1674) (8.458, 41.1587) (8.4531, 41.1501) (8.4481, 41.1415) (8.4432, 41.133) (8.4384, 41.1244) (8.4335, 41.116) (8.4287, 41.1075) (8.4239, 41.0991) (8.4192, 41.0907) (8.4145, 41.0823) (8.4098, 41.074) (8.4052, 41.0657) (8.4006, 41.0574) (8.396, 41.0491) (8.3915, 41.0409) (8.387, 41.0328) (8.3825, 41.0246) (8.3781, 41.0165) (8.3737, 41.0085) (8.3693, 41.0004) (8.365, 40.9924) (8.3607, 40.9845) (8.3565, 40.9765) (8.3522, 40.9686) (8.348, 40.9608) (8.3439, 40.9529) (8.3398, 40.9452) (8.3357, 40.9374) (8.3316, 40.9297) (8.3276, 40.922) (8.3236, 40.9144) (8.3196, 40.9068) (8.3157, 40.8992) (8.3118, 40.8917) (8.308, 40.8842) (8.3042, 40.8767) (8.3004, 40.8693) (8.2966, 40.8619) (8.2929, 40.8546) (8.2892, 40.8473) (8.2856, 40.8401) (8.282, 40.8329) (8.2784, 40.8257) (8.2748, 40.8186) (8.2713, 40.8115) (8.2678, 40.8044) (8.2644, 40.7974) (8.261, 40.7905) (8.2576, 40.7835) (8.2543, 40.7767) (8.251, 40.7698) (8.2477, 40.763) (8.2445, 40.7563) (8.2412, 40.7496) (8.2381, 40.7429) (8.2349, 40.7363) (8.2318, 40.7298) (8.2288, 40.7233) (8.2257, 40.7168) (8.2227, 40.7104) (8.2198, 40.704) (8.2169, 40.6977) (8.214, 40.6914) (8.2111, 40.6851) (8.2083, 40.679) (8.2055, 40.6728) (8.2027, 40.6667) (8.2, 40.6607) (8.1973, 40.6547) (8.1947, 40.6488) (8.192, 40.6429) (8.1895, 40.6371) (8.1869, 40.6313) (8.1844, 40.6256) (8.1819, 40.6199) (8.1795, 40.6143) (8.177, 40.6087) (8.1747, 40.6032) (8.1723, 40.5978) (8.17, 40.5924) (8.1677, 40.587) (8.1655, 40.5818) (8.1633, 40.5765) (8.1611, 40.5714) (8.159, 40.5663) (8.1569, 40.5612) (8.1548, 40.5562) (8.1528, 40.5513) (8.1508, 40.5464) (8.1488, 40.5416) (8.1469, 40.5369) (8.145, 40.5322) (8.1432, 40.5276) (8.1413, 40.523) (8.1395, 40.5185) (8.1378, 40.5141) (8.1361, 40.5097) (8.1344, 40.5054) (8.1327, 40.5012) (8.1311, 40.497) (8.1295, 40.4929) (8.128, 40.4889) (8.1265, 40.4849) (8.125, 40.4811) (8.1236, 40.4772) (8.1222, 40.4735) (8.1208, 40.4698) (8.1194, 40.4662) (8.1181, 40.4627) (8.1169, 40.4593) (8.1156, 40.4559) (8.1144, 40.4526) (8.1133, 40.4494) (8.1121, 40.4462) (8.1111, 40.4432) (8.11, 40.4402) (8.109, 40.4373) (8.108, 40.4345) (8.107, 40.4318) (8.1061, 40.4291) (8.1052, 40.4265) (8.1044, 40.4241) (8.1036, 40.4217) (8.1028, 40.4194) (8.102, 40.4172) (8.1013, 40.415) (8.1007, 40.413) (8.1, 40.4111) (8.0994, 40.4092) (8.0988, 40.4075) (8.0983, 40.4058) (8.0978, 40.4043) (8.0973, 40.4028) (8.0969, 40.4015) (8.0965, 40.4002) (8.0962, 40.3991) (8.0958, 40.398) (8.0956, 40.3971) (8.0953, 40.3963) (8.0951, 40.3956) (8.0949, 40.3951) (8.0948, 40.3948) (8.0948, 40.3946) (8.0948, 40.3945) knots -1 -1 -1 -1 -1 -1 -0.99583333 -0.99166667 -0.9875 -0.98333333 -0.97916667 -0.975 -0.97083333 -0.96666667 -0.9625 -0.95833333 -0.95416667 -0.95 -0.94583333 -0.94166667 -0.9375 -0.93333333 -0.92916667 -0.925 -0.92083333 -0.91666667 -0.9125 -0.90833333 -0.90416667 -0.9 -0.89583333 -0.89166667 -0.8875 -0.88333333 -0.87916667 -0.875 -0.87083333 -0.86666667 -0.8625 -0.85833333 -0.85416667 -0.85 -0.84583333 -0.84166667 -0.8375 -0.83333333 -0.82916667 -0.825 -0.82083333 -0.81666667 -0.8125 -0.80833333 -0.80416667 -0.8 -0.79583333 -0.79166667 -0.7875 -0.78333333 -0.77916667 -0.775 -0.77083333 -0.76666667 -0.7625 -0.75833333 -0.75416667 -0.75 -0.74583333 -0.74166667 -0.7375 -0.73333333 -0.72916667 -0.725 -0.72083333 -0.71666667 -0.7125 -0.70833333 -0.70416667 -0.7 -0.69583333 -0.69166667 -0.6875 -0.68333333 -0.67916667 -0.675 -0.67083333 -0.66666667 -0.6625 -0.65833333 -0.65416667 -0.65 -0.64583333 -0.64166667 -0.6375 -0.63333333 -0.62916667 -0.625 -0.62083333 -0.61666667 -0.6125 -0.60833333 -0.60416667 -0.6 -0.59583333 -0.59166667 -0.5875 -0.58333333 -0.57916667 -0.575 -0.57083333 -0.56666667 -0.5625 -0.55833333 -0.55416667 -0.55 -0.54583333 -0.54166667 -0.5375 -0.53333333 -0.52916667 -0.525 -0.52083333 -0.51666667 -0.5125 -0.50833333 -0.50416667 -0.5 -0.49583333 -0.49166667 -0.4875 -0.48333333 -0.47916667 -0.475 -0.47083333 -0.46666667 -0.4625 -0.45833333 -0.45416667 -0.45 -0.44583333 -0.44166667 -0.4375 -0.43333333 -0.42916667 -0.425 -0.42083333 -0.41666667 -0.4125 -0.40833333 -0.40416667 -0.4 -0.39583333 -0.39166667 -0.3875 -0.38333333 -0.37916667 -0.375 -0.37083333 -0.36666667 -0.3625 -0.35833333 -0.35416667 -0.35 -0.34583333 -0.34166667 -0.3375 -0.33333333 -0.32916667 -0.325 -0.32083333 -0.31666667 -0.3125 -0.30833333 -0.30416667 -0.3 -0.29583333 -0.29166667 -0.2875 -0.28333333 -0.27916667 -0.275 -0.27083333 -0.26666667 -0.2625 -0.25833333 -0.25416667 -0.25 -0.24583333 -0.24166667 -0.2375 -0.23333333 -0.22916667 -0.225 -0.22083333 -0.21666667 -0.2125 -0.20833333 -0.20416667 -0.2 -0.19583333 -0.19166667 -0.1875 -0.18333333 -0.17916667 -0.175 -0.17083333 -0.16666667 -0.1625 -0.15833333 -0.15416667 -0.15 -0.14583333 -0.14166667 -0.1375 -0.13333333 -0.12916667 -0.125 -0.12083333 -0.11666667 -0.1125 -0.10833333 -0.10416667 -0.1 -0.09583333 -0.09166667 -0.0875 -0.08333333 -0.07916667 -0.075 -0.07083333 -0.06666667 -0.0625 -0.05833333 -0.05416667 -0.05 -0.04583333 -0.04166667 -0.0375 -0.03333333 -0.02916667 -0.025 -0.02083333 -0.01666667 -0.0125 -0.00833333 -0.00416667 0 0 0 0 0 0
  spline S118 degree 5 poles (12.6495, 38.6461) (12.6495, 38.6462) (12.6496, 38.6464) (12.6497, 38.6467) (12.65, 38.6471) (12.6503, 38.6478) (12.6506, 38.6486) (12.651, 38.6495) (12.6515, 38.6504) (12.652, 38.6515) (12.6526, 38.6527) (12.6531, 38.654) (12.6538, 38.6554) (12.6544, 38.6569) (12.6551, 38.6585) (12.6559, 38.6602) (12.6567, 38.6619) (12.6575, 38.6638) (12.6583, 38.6658) (12.6592, 38.6678) (12.6602, 38.67) (12.6611, 38.6722) (12.6621, 38.6745) (12.6631, 38.6769) (12.6642, 38.6794) (12.6653, 38.682) (12.6664, 38.6847) (12.6676, 38.6874) (12.6687, 38.6903) (12.6699, 38.6932) (12.6712, 38.6962) (12.6724, 38.6993) (12.6737, 38.7024) (12.675, 38.7057) (12.6764, 38.709) (12.6778, 38.7124) (12.6791, 38.7159) (12.6806, 38.7195) (12.682, 38.7231) (12.6834, 38.7269) (12.6849, 38.7307) (12.6864, 38.7345) (12.688, 38.7385) (12.6895, 38.7425) (12.6911, 38.7466) (12.6927, 38.7508) (12.6943, 38.755) (12.6959, 38.7594) (12.6975, 38.7638) (12.6992, 38.7682) (12.7009, 38.7728) (12.7026, 38.7774) (12.7043, 38.782) (12.706, 38.7868) (12.7077, 38.7916) (12.7095, 38.7965) (12.7113, 38.8015) (12.7131, 38.8065) (12.7149, 38.8116) (12.7167, 38.8167) (12.7185, 38.822) (12.7204, 38.8273) (12.7222, 38.8326) (12.7241, 38.838) (12.726, 38.8435) (12.7279, 38.8491) (12.7298, 38.8547) (12.7317, 38.8604) (12.7336, 38.8661) (12.7356, 38.8719) (12.7375, 38.8778) (12.7395, 38.8837) (12.7414, 38.8897) (12.7434, 38.8958) (12.7454, 38.9019) (12.7474, 38.9081) (12.7494, 38.9144) (12.7514, 38.9207) (12.7534, 38.927) (12.7555, 38.9335) (12.7575, 38.9399) (12.7596, 38.9465) (12.7616, 38.9531) (12.7637, 38.9598) (12.7657, 38.9665) (12.7678, 38.9733) (12.7699, 38.9801) (12.772, 38.987) (12.774, 38.9939) (12.7761, 39.0009) (12.7782, 39.008) (12.7803, 39.0151) (12.7824, 39.0223) (12.7845, 39.0296) (12.7867, 39.0368) (12.7888, 39.0442) (12.7909, 39.0516) (12.793, 39.059) (12.7952, 39.0665) (12.7973, 39.0741) (12.7994, 39.0817) (12.8016, 39.0894) (12.8037, 39.0971) (12.8058, 39.1049) (12.808, 39.1127) (12.8101, 39.1206) (12.8123, 39.1286) (12.8144, 39.1365) (12.8166, 39.1446) (12.8187, 39.1527) (12.8208, 39.1608) (12.823, 39.169) (12.8251, 39.1773) (12.8273, 39.1856) (12.8294, 39.1939) (12.8316, 39.2023) (12.8337, 39.2108) (12.8359, 39.2193) (12.838, 39.2278) (12.8402, 39.2364) (12.8423, 39.2451) (12.8445, 39.2537) (12.8466, 39.2625) (12.8487, 39.2713) (12.8509, 39.2801) (12.853, 39.289) (12.8551, 39.298) (12.8573, 39.3069) (12.8594, 39.316) (12.8615, 39.3251) (12.8636, 39.3342) (12.8658, 39.3434) (12.8679, 39.3526) (12.87, 39.3619) (12.8721, 39.3712) (12.8742, 39.3806) (12.8763, 39.39) (12.8784, 39.3994) (12.8805, 39.4089) (12.8826, 39.4185) (12.8847, 39.4281) (12.8867, 39.4377) (12.8888, 39.4474) (12.8909, 39.4571) (12.8929, 39.4669) (12.895, 39.4767) (12.8971, 39.4866) (12.8991, 39.4965) (12.9011, 39.5064) (12.9032, 39.5164) (12.9052, 39.5265) (12.9072, 39.5365) (12.9093, 39.5467) (12.9113, 39.5568) (12.9133, 39.5671) (12.9153, 39.5773) (12.9173, 39.5876) (12.9193, 39.5979) (12.9213, 39.6083) (12.9232, 39.6188) (12.9252, 39.6292) (12.9272, 39.6397) (12.9291, 39.6503) (12.9311, 39.6609) (12.933, 39.6715) (12.9349, 39.6822) (12.9368, 39.6929) (12.9388, 39.7037) (12.9407, 39.7145) (12.9426, 39.7253) (12.9445, 39.7362) (12.9463, 39.7471) (12.9482, 39.7581) (12.9501, 39.7691) (12.9519, 39.7801) (12.9538, 39.7912) (12.9556, 39.8023) (12.9574, 39.8135) (12.9593, 39.8247) (12.9611, 39.8359) (12.9629, 39.8472) (12.9647, 39.8585) (12.9665, 39.8699) (12.9682, 39.8813) (12.97, 39.8927) (12.9718, 39.9042) (12.9735, 39.9157) (12.9752, 39.9273) (12.977, 39.9388) (12.9787, 39.9505) (12.9804, 39.9621) (12.9821, 39.9738) (12.9838, 39.9856) (12.9854, 39.9974) (12.9871, 40.0092) (12.9887, 40.021) (12.9904, 40.0329) (12.992, 40.0449) (12.9936, 40.0568) (12.9952, 40.0688) (12.9968, 40.0809) (12.9984, 40.0929) (13, 40.105) (13.0016, 40.1172) (13.0031, 40.1294) (13.0047, 40.1416) (13.0062, 40.1539) (13.0077, 40.1661) (13.0092, 40.1785) (13.0107, 40.1908) (13.0122, 40.2032) (13.0136, 40.2157) (13.0151, 40.2281) (13.0165, 40.2406) (13.018, 40.2532) (13.0194, 40.2658) (13.0208, 40.2784) (13.0222, 40.291) (13.0236, 40.3037) (13.0249, 40.3164) (13.0263, 40.3291) (13.0276, 40.3419) (13.029, 40.3547) (13.0303, 40.3676) (13.0316, 40.3805) (13.0329, 40.3934) (13.0342, 40.4063) (13.0354, 40.4193) (13.0367, 40.4323) (13.0379, 40.4454) (13.0391, 40.4585) (13.0404, 40.4716) (13.0415, 40.4848) (13.0427, 40.4979) (13.0439, 40.5112) (13.0451, 40.5244) (13.0462, 40.5377) (13.0473, 40.551) (13.0484, 40.5644) (13.0495, 40.5777) (13.0506, 40.5911) (13.0515, 40.6019) (13.0521, 40.61) (13.0525, 40.6154) (13.0527, 40.6181) knots 0 0 0 0 0 0 0.00416667 0.00833333 0.0125 0.01666667 0.02083333 0.025 0.02916667 0.03333333 0.0375 0.04166667 0.04583333 0.05 0.05416667 0.05833333 0.0625 0.06666667 0.07083333 0.075 0.07916667 0.08333333 0.0875 0.09166667 0.09583333 0.1 0.10416667 0.10833333 0.1125 0.11666667 0.12083333 0.125 0.12916667 0.13333333 0.1375 0.14166667 0.14583333 0.15 0.15416667 0.15833333 0.1625 0.16666667 0.17083333 0.175 0.17916667 0.18333333 0.1875 0.19166667 0.19583333 0.2 0.20416667 0.20833333 0.2125 0.21666667 0.22083333 0.225 0.22916667 0.23333333 0.2375 0.24166667 0.24583333 0.25 0.25416667 0.25833333 0.2625 0.26666667 0.27083333 0.275 0.27916667 0.28333333 0.2875 0.29166667 0.29583333 0.3 0.30416667 0.30833333 0.3125 0.31666667 0.32083333 0.325 0.32916667 0.33333333 0.3375 0.34166667 0.34583333 0.35 0.35416667 0.35833333 0.3625 0.36666667 0.37083333 0.375 0.37916667 0.38333333 0.3875 0.39166667 0.39583333 0.4 0.40416667 0.40833333 0.4125 0.41666667 0.42083333 0.425 0.42916667 0.43333333 0.4375 0.44166667 0.44583333 0.45 0.45416667 0.45833333 0.4625 0.46666667 0.47083333 0.475 0.47916667 0.48333333 0.4875 0.49166667 0.49583333 0.5 0.50416667 0.50833333 0.5125 0.51666667 0.52083333 0.525 0.52916667 0.53333333 0.5375 0.54166667 0.54583333 0.55 0.55416667 0.55833333 0.5625 0.56666667 0.57083333 0.575 0.57916667 0.58333333 0.5875 0.59166667 0.59583333 0.6 0.60416667 0.60833333 0.6125 0.61666667 0.62083333 0.625 0.62916667 0.63333333 0.6375 0.64166667 0.64583333 0.65 0.65416667 0.65833333 0.6625 0.66666667 0.67083333 0.675 0.67916667 0.68333333 0.6875 0.69166667 0.69583333 0.7 0.70416667 0.70833333 0.7125 0.71666667 0.72083333 0.725 0.72916667 0.73333333 0.7375 0.74166667 0.74583333 0.75 0.75416667 0.75833333 0.7625 0.76666667 0.77083333 0.775 0.77916667 0.78333333 0.7875 0.79166667 0.79583333 0.8 0.80416667 0.80833333 0.8125 0.81666667 0.82083333 0.825 0.82916667 0.83333333 0.8375 0.84166667 0.84583333 0.85 0.85416667 0.85833333 0.8625 0.86666667 0.87083333 0.875 0.87916667 0.88333333 0.8875 0.89166667 0.89583333 0.9 0.90416667 0.90833333 0.9125 0.91666667 0.92083333 0.925 0.92916667 0.93333333 0.9375 0.94166667 0.94583333 0.95 0.95416667 0.95833333 0.9625 0.96666667 0.97083333 0.975 0.97916667 0.98333333 0.9875 0.99166667 0.99583333 1 1 1 1 1 1
  line L246 (27.8945, 4.4052) -> (27.8937, 4.4055)
  spline S119 degree 5 poles (9.8472, 39.8251) (9.8472, 39.8252) (9.8473, 39.8254) (9.8474, 39.8257) (9.8475, 39.8262) (9.8478, 39.8269) (9.8481, 39.8277) (9.8484, 39.8286) (9.8487, 39.8296) (9.8491, 39.8308) (9.8495, 39.832) (9.85, 39.8334) (9.8505, 39.8348) (9.851, 39.8364) (9.8515, 39.838) (9.8521, 39.8398) (9.8527, 39.8416) (9.8533, 39.8435) (9.8539, 39.8456) (9.8546, 39.8477) (9.8553, 39.8499) (9.856, 39.8523) (9.8568, 39.8547) (9.8575, 39.8572) (9.8583, 39.8598) (9.8591, 39.8625) (9.86, 39.8652) (9.8608, 39.8681) (9.8617, 39.871) (9.8626, 39.8741) (9.8635, 39.8772) (9.8645, 39.8804) (9.8654, 39.8837) (9.8664, 39.887) (9.8674, 39.8905) (9.8684, 39.894) (9.8694, 39.8976) (9.8704, 39.9013) (9.8715, 39.9051) (9.8725, 39.909) (9.8736, 39.9129) (9.8747, 39.9169) (9.8758, 39.921) (9.8769, 39.9252) (9.878, 39.9294) (9.8792, 39.9337) (9.8803, 39.9381) (9.8815, 39.9426) (9.8827, 39.9471) (9.8838, 39.9517) (9.885, 39.9564) (9.8862, 39.9612) (9.8874, 39.966) (9.8887, 39.9709) (9.8899, 39.9759) (9.8911, 39.981) (9.8924, 39.9861) (9.8936, 39.9912) (9.8949, 39.9965) (9.8962, 40.0018) (9.8974, 40.0072) (9.8987, 40.0127) (9.9, 40.0182) (9.9013, 40.0238) (9.9026, 40.0294) (9.9039, 40.0352) (9.9052, 40.0409) (9.9065, 40.0468) (9.9079, 40.0527) (9.9092, 40.0587) (9.9105, 40.0647) (9.9118, 40.0709) (9.9132, 40.077) (9.9145, 40.0833) (9.9158, 40.0896) (9.9172, 40.0959) (9.9185, 40.1023) (9.9199, 40.1088) (9.9212, 40.1154) (9.9225, 40.122) (9.9239, 40.1286) (9.9252, 40.1353) (9.9266, 40.1421) (9.9279, 40.149) (9.9293, 40.1559) (9.9306, 40.1628) (9.932, 40.1698) (9.9333, 40.1769) (9.9347, 40.1841) (9.936, 40.1912) (9.9374, 40.1985) (9.9387, 40.2058) (9.9401, 40.2132) (9.9414, 40.2206) (9.9428, 40.228) (9.9441, 40.2356) (9.9454, 40.2431) (9.9468, 40.2508) (9.9481, 40.2585) (9.9494, 40.2662) (9.9508, 40.274) (9.9521, 40.2819) (9.9534, 40.2898) (9.9547, 40.2977) (9.956, 40.3057) (9.9573, 40.3138) (9.9586, 40.3219) (9.9599, 40.3301) (9.9612, 40.3383) (9.9625, 40.3466) (9.9638, 40.3549) (9.9651, 40.3633) (9.9664, 40.3717) (9.9676, 40.3802) (9.9689, 40.3887) (9.9701, 40.3973) (9.9714, 40.4059) (9.9726, 40.4146) (9.9739, 40.4233) (9.9751, 40.4321) (9.9763, 40.4409) (9.9776, 40.4498) (9.9788, 40.4587) (9.98, 40.4677) (9.9812, 40.4767) (9.9824, 40.4858) (9.9836, 40.4949) (9.9847, 40.504) (9.9859, 40.5133) (9.9871, 40.5225) (9.9882, 40.5318) (9.9894, 40.5412) (9.9905, 40.5506) (9.9916, 40.56) (9.9928, 40.5695) (9.9939, 40.579) (9.995, 40.5886) (9.9961, 40.5982) (9.9972, 40.6079) (9.9983, 40.6176) (9.9993, 40.6274) (10.0004, 40.6372) (10.0014, 40.647) (10.0025, 40.6569) (10.0035, 40.6668) (10.0045, 40.6768) (10.0055, 40.6868) (10.0065, 40.6969) (10.0075, 40.707) (10.0085, 40.7172) (10.0095, 40.7274) (10.0104, 40.7376) (10.0114, 40.7479) (10.0123, 40.7582) (10.0133, 40.7686) (10.0142, 40.779) (10.0151, 40.7894) (10.016, 40.7999) (10.0169, 40.8105) (10.0177, 40.821) (10.0186, 40.8317) (10.0195, 40.8423) (10.0203, 40.853) (10.0211, 40.8638) (10.0219, 40.8745) (10.0227, 40.8854) (10.0235, 40.8962) (10.0243, 40.9071) (10.0251, 40.9181) (10.0258, 40.929) (10.0266, 40.94) (10.0273, 40.9511) (10.028, 40.9622) (10.0287, 40.9733) (10.0294, 40.9845) (10.0301, 40.9957) (10.0308, 41.007) (10.0314, 41.0183) (10.0321, 41.0296) (10.0327, 41.041) (10.0333, 41.0524) (10.0339, 41.0638) (10.0345, 41.0753) (10.0351, 41.0868) (10.0356, 41.0984) (10.0362, 41.11) (10.0367, 41.1216) (10.0372, 41.1333) (10.0377, 41.145) (10.0382, 41.1567) (10.0387, 41.1685) (10.0392, 41.1803) (10.0396, 41.1922) (10.04, 41.2041) (10.0405, 41.216) (10.0409, 41.228) (10.0412, 41.24) (10.0416, 41.252) (10.042, 41.2641) (10.0423, 41.2762) (10.0427, 41.2883) (10.043, 41.3005) (10.0433, 41.3127) (10.0436, 41.3249) (10.0438, 41.3372) (10.0441, 41.3495) (10.0443, 41.3619) (10.0445, 41.3743) (10.0448, 41.3867) (10.0449, 41.3991) (10.0451, 41.4116) (10.0453, 41.4241) (10.0454, 41.4367) (10.0456, 41.4493) (10.0457, 41.4619) (10.0458, 41.4745) (10.0458, 41.4872) (10.0459, 41.5) (10.046, 41.5127) (10.046, 41.5255) (10.046, 41.5383) (10.046, 41.5512) (10.046, 41.5641) (10.046, 41.577) (10.0459, 41.5899) (10.0458, 41.6029) (10.0458, 41.6159) (10.0457, 41.629) (10.0455, 41.642) (10.0454, 41.6551) (10.0453, 41.6683) (10.0451, 41.6815) (10.0449, 41.6947) (10.0447, 41.7079) (10.0445, 41.7212) (10.0442, 41.7345) (10.044, 41.7478) (10.0437, 41.7612) (10.0434, 41.7745) (10.0431, 41.788) (10.0428, 41.8014) (10.0425, 41.8122) (10.0423, 41.8203) (10.0422, 41.8257) (10.0421, 41.8284) knots 0 0 0 0 0 0 0.00416667 0.00833333 0.0125 0.01666667 0.02083333 0.025 0.02916667 0.03333333 0.0375 0.04166667 0.04583333 0.05 0.05416667 0.05833333 0.0625 0.06666667 0.07083333 0.075 0.07916667 0.08333333 0.0875 0.09166667 0.09583333 0.1 0.10416667 0.10833333 0.1125 0.11666667 0.12083333 0.125 0.12916667 0.13333333 0.1375 0.14166667 0.14583333 0.15 0.15416667 0.15833333 0.1625 0.16666667 0.17083333 0.175 0.17916667 0.18333333 0.1875 0.19166667 0.19583333 0.2 0.20416667 0.20833333 0.2125 0.21666667 0.22083333 0.225 0.22916667 0.23333333 0.2375 0.24166667 0.24583333 0.25 0.25416667 0.25833333 0.2625 0.26666667 0.27083333 0.275 0.27916667 0.28333333 0.2875 0.29166667 0.29583333 0.3 0.30416667 0.30833333 0.3125 0.31666667 0.32083333 0.325 0.32916667 0.33333333 0.3375 0.34166667 0.34583333 0.35 0.35416667 0.35833333 0.3625 0.36666667 0.37083333 0.375 0.37916667 0.38333333 0.3875 0.39166667 0.39583333 0.4 0.40416667 0.40833333 0.4125 0.41666667 0.42083333 0.425 0.42916667 0.43333333 0.4375 0.44166667 0.44583333 0.45 0.45416667 0.45833333 0.4625 0.46666667 0.47083333 0.475 0.47916667 0.48333333 0.4875 0.49166667 0.49583333 0.5 0.50416667 0.50833333 0.5125 0.51666667 0.52083333 0.525 0.52916667 0.53333333 0.5375 0.54166667 0.54583333 0.55 0.55416667 0.55833333 0.5625 0.56666667 0.57083333 0.575 0.57916667 0.58333333 0.5875 0.59166667 0.59583333 0.6 0.60416667 0.60833333 0.6125 0.61666667 0.62083333 0.625 0.62916667 0.63333333 0.6375 0.64166667 0.64583333 0.65 0.65416667 0.65833333 0.6625 0.66666667 0.67083333 0.675 0.67916667 0.68333333 0.6875 0.69166667 0.69583333 0.7 0.70416667 0.70833333 0.7125 0.71666667 0.72083333 0.725 0.72916667 0.73333333 0.7375 0.74166667 0.74583333 0.75 0.75416667 0.75833333 0.7625 0.76666667 0.77083333 0.775 0.77916667 0.78333333 0.7875 0.79166667 0.79583333 0.8 0.80416667 0.80833333 0.8125 0.81666667 0.82083333 0.825 0.82916667 0.83333333 0.8375 0.84166667 0.84583333 0.85 0.85416667 0.85833333 0.8625 0.86666667 0.87083333 0.875 0.87916667 0.88333333 0.8875 0.89166667 0.89583333 0.9 0.90416667 0.90833333 0.9125 0.91666667 0.92083333 0.925 0.92916667 0.93333333 0.9375 0.94166667 0.94583333 0.95 0.95416667 0.95833333 0.9625 0.96666667 0.97083333 0.975 0.97916667 0.98333333 0.9875 0.99166667 0.99583333 1 1 1 1 1 1
  line L247 (28.7753, 16.4508) -> (28.7745, 16.4507)
  line L248 (18.7401, 34.6898) -> (18.5501, 34.4649)
  arc A125 (-2.0967, -16.1734) -> (-0.9119, -16.2355) centre (0, 12.5) ccw
  arc A126 (28.4828, 16.4106) -> (28.2972, 17.5824) centre (0, 12.5) ccw
  line L249 (28.7745, 16.4507) -> (28.4828, 16.4106)
  line L250 (28.2972, 17.5824) -> (28.587, 17.6345)
  line L251 (27.918, 5.6335) -> (28.2039, 5.5632)
  arc A127 (30.8773, 15.255) -> (30.7754, 16.2249) centre (0, 12.5) ccw
  arc A128 (9.1146, -17.1298) -> (10.0421, -16.8284) centre (0, 12.5) ccw
  arc A129 (6.9214, 42.7174) -> (5.9675, 42.9202) centre (0, 12.5) ccw
  line L252 (3.9106, 40.9828) -> (3.9507, 41.2745)
  arc A130 (6.8665, -15.418) -> (8.0125, -15.1109) centre (0, 12.5) ccw
  line L253 (19, 25) -> (25.8803, 25.0209)
  line L254 (-19, 25) -> (-25.8803, 25.0209)
  point P0 (0, 12.5)
  constraint coincident L3.end L4.start
  constraint coincident L10.end L11.start